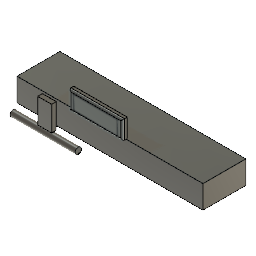
AIR MONITORING SYSTEM (Autodesk Fusion 360 design; units mm, degrees)
part number: 2025-06-21-12-44-40-260
part number: 2025-06-22-20-37-10-976
Autodesk Fusion 360 part; units mm, degrees
sketch "Sketch1" plane through (0, 0, 0) normal (1, 0, 0) x (0, 1, 0) in component "power supply"
  circle A0 centre (0, 0) radius 69.6419
  dimension "d1" = 139.2839
  constraint coincident A0.centre origin
  measures "d1" diameter of A0
extrude "Extrude1" add sketch "Sketch1" along normal blind 1400 makes body 1 in component "power supply"
sketch "Sketch2" plane through (1400, 0, 0) normal (1, 0, 0) x (0, 1, 0) in component "power supply"
  circle A0 centre (0, 0) radius 69.6419
sketch "Sketch3" plane through (0, 0, 0) normal (0, 0, 1) x (1, 0, 0) in component "power supply"
  line L0 (850, 50) -> (850, -23.9285)
  line L1 (850, -23.9285) -> (550, -23.9285)
  line L2 (550, -23.9285) -> (550, 50)
  line L3 (550, 50) -> (850, 50)
  dimension "d4" = 300
  dimension "d5" = 73.9285
  dimension "d6" = 550
  dimension "d7" = 23.9285
  constraint perpendicular L0 L1
  constraint parallel L0 L2
  constraint parallel L1 L3
  constraint vertical L0
  measures "d4" distance of L0 L2
  measures "d5" distance of L1 L3
  measures "d6" distance of origin L2
  measures "d7" distance of origin L1
extrude "Extrude2" cut sketch "Sketch3" along normal blind 3000 bodies 1 in component "power supply"
sketch "Sketch4" plane through (0, -23.9285, 0) normal (0, 1, 0) x (-1, 0, 0) in component "power supply"
  line L0 (-550, 65.4021) -> (-850, 65.4021)
  line L1 (-850, 65.4021) -> (-850, 0)
  line L2 (-850, 0) -> (-550, 0)
  line L3 (-550, 0) -> (-550, 65.4021)
  line L4 (-850, 65.4021) -> (-850, 600)
  line L5 (-850, 600) -> (-550, 600)
  line L6 (-550, 600) -> (-550, 65.4021)
  line L7 (-550, 65.4021) -> (-850, 65.4021)
  dimension "d10" = 600
  constraint perpendicular L4 L5
  constraint parallel L4 L6
  constraint parallel L5 L7
  constraint perpendicular L0 L4
  constraint coincident L0.end L1.start
  constraint collinear L3 L6
  measures "d10" distance of L2 L5
extrude "Extrude3" add sketch "Sketch4" along normal blind 100 separate body contours L0 L4 L5 L6 L7 makes body 2 in component "power supply"
sketch "Sketch5" plane through (0, 0, 0) normal (1, 0, 0) x (0, 1, 0) in component "power supply"
  line L0 (76.99, 152.1023) -> (76.99, 650)
  line L1 (76.99, 650) -> (1000.8704, 650)
  line L2 (1000.8704, 650) -> (1000.8704, 152.1023)
  line L3 (1000.8704, 152.1023) -> (76.99, 152.1023)
  dimension "d13" = 923.8804
  dimension "d14" = 497.8977
  dimension "d15" = 76.99
  dimension "d16" = 152.1023
  constraint perpendicular L0 L1
  constraint parallel L0 L2
  constraint parallel L1 L3
  constraint vertical L0
  measures "d13" distance of L0 L2
  measures "d14" distance of L1 L3
  measures "d15" distance of origin L0
  measures "d16" distance of origin L3
extrude "Extrude4" add sketch "Sketch5" along normal blind 4000 separate body makes body 3 in component "power supply"
sketch "Sketch6" plane through (0, 0, 0) normal (0, 1, 0) x (1, 0, 0) in component "power supply"
  line L0 (1398.3055, 59.0819) -> (1398.3055, 700)
  line L1 (1398.3055, 700) -> (1.7504, 700)
  line L2 (1.7504, 700) -> (1.7504, 59.0819)
  line L3 (1.7504, 59.0819) -> (1398.3055, 59.0819)
  dimension "d19" = 1396.5551
  dimension "d20" = 640.9181
  dimension "d21" = 1.7504
  dimension "d22" = 59.0819
  constraint perpendicular L0 L1
  constraint parallel L0 L2
  constraint parallel L1 L3
  constraint vertical L0
  measures "d19" distance of L0 L2
  measures "d20" distance of L1 L3
  measures "d21" distance of origin L2
  measures "d22" distance of origin L3
extrude "Extrude5" cut sketch "Sketch6" along normal blind 80 bodies 1 in component "power supply"
sketch "Sketch7" plane through (0, 0, 0) normal (0, 1, 0) x (1, 0, 0) in component "power supply"
  line L0 (1393.7184, 54.9495) -> (1393.7184, 600)
  line L1 (1393.7184, 600) -> (0, 600)
  line L2 (0, 600) -> (0, 54.9495)
  line L3 (0, 54.9495) -> (1393.7184, 54.9495)
  dimension "d25" = 1393.7184
  dimension "d26" = 545.0505
  dimension "d27" = 54.9495
  constraint perpendicular L0 L1
  constraint parallel L0 L2
  constraint parallel L1 L3
  constraint vertical L0
  constraint vertical origin L2.end
  measures "d25" distance of L0 L2
  measures "d26" distance of L1 L3
  measures "d27" distance of origin L3
extrude "Extrude6" cut sketch "Sketch7" along normal blind 60 bodies 1 in component "power supply"
sketch "Sketch1 (2)" plane through (0, 0, 650) normal (0, 0, 1) x (-1, 0, 0)
  line L0 (0, -1000.8704) -> (0, -76.99)
  line L1 (0, -76.99) -> (-4000, -76.99)
  line L2 (-4000, -76.99) -> (-4000, -1000.8704)
  line L3 (-4000, -1000.8704) -> (0, -1000.8704)
sketch "Sketch8" plane through (0, 0, 0) normal (0, 1, 0) x (1, 0, 0) in component "power supply"
  line L0 (1200, -650) -> (1200, -1050)
  line L1 (1200, -1050) -> (2350, -1050)
  line L2 (2350, -1050) -> (2350, -650)
  line L3 (2350, -650) -> (1200, -650)
  dimension "d30" = 1150
  dimension "d31" = 400
  dimension "d32" = 1200
  dimension "d33" = 650
  constraint perpendicular L0 L1
  constraint parallel L0 L2
  constraint parallel L1 L3
  constraint vertical L0
  measures "d30" distance of L0 L2
  measures "d31" distance of L1 L3
  measures "d32" distance of origin L0
  measures "d33" distance of origin L3
extrude "Extrude7" add sketch "Sketch8" along normal blind 100 bodies 3 in component "power supply"
sketch "Sketch9" plane through (0, 0, 0) normal (0, -1, 0) x (1, 0, 0) in component "power supply"
  line L0 (1200, 650) -> (2350, 650)
  line L1 (2350, 650) -> (2350, 1050)
  line L2 (2350, 1050) -> (1200, 1050)
  line L3 (1200, 1050) -> (1200, 650)
  line L4 (1300, 1000) -> (1300, 700)
  line L5 (1300, 700) -> (2238.5709, 700)
  line L6 (2238.5709, 700) -> (2238.5709, 1000)
  line L7 (2238.5709, 1000) -> (1300, 1000)
  dimension "d36" = 300
  dimension "d37" = 938.5709
  dimension "d38" = 100
  dimension "d39" = 50
  constraint perpendicular L4 L5
  constraint parallel L4 L6
  constraint parallel L5 L7
  constraint parallel L3 L4
  measures "d36" distance of L5 L7
  measures "d37" distance of L4 L6
  measures "d38" distance of L3 L4
  measures "d39" distance of L0 L5
fillet "Fillet1" radius 40 1 faces at (1583.3333, 0, 783.3333) on bodies 3 in component "power supply"
sketch "Sketch2 (2)" plane through (0, 0, 650) normal (0, 0, 1) x (-1, 0, 0)
component "power supply" placed x (1, 0, 0) y (0, 1, 0) z (0, 0, 1) at (0, 0, 0)
